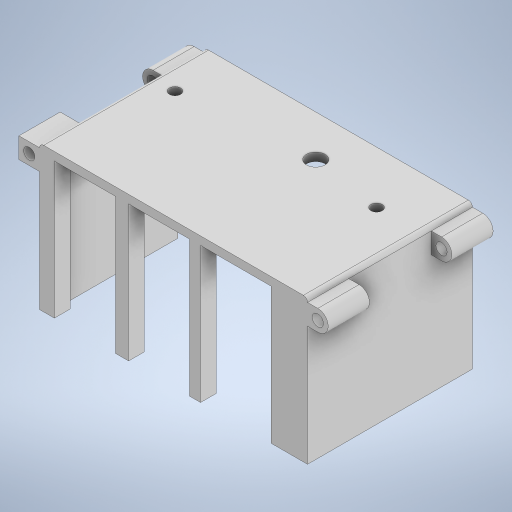
# Autodesk Inventor part: TOTAL
Saved by Autodesk Inventor 2023.1 (Build 271208000, 208)
## iProperties
Created: 2023-01-22
Part Number: TOTAL
Material: Generic
Document SubType Name: Modeling
Designer: liaar
Density: 1 g/cm^3
Appearance: Default
Author: liaar
Autodesk Inventor part; units mm, degrees
sketch "Sketch1" plane through (0, 0, 0) normal (0, 1, 0) x (-1, 0, 0)
  line L0 (0, 0) -> (-65, 0)
  line L1 (-65, 0) -> (-65, -121.25)
  line L2 (-65, -121.25) -> (0, -121.25)
  line L3 (0, -121.25) -> (0, 0)
  dimension "d0" = 121.25
  dimension "d1" = 65
  constraints: 8 end point, 2 parallel, 1 horizontal, 1 perpendicular
  measures "d0" distance of L0.end L1.end
  measures "d1" distance of L1.end L2.end
extrude "Extrusion1" add sketch "Sketch1" against normal blind 35
sketch "Sketch2" plane through (0, 0, 0) normal (0, 1, 0) x (1, 0, 0)
  line L0 (0, 0) -> (65, 0) projected
  line L1 (0, 121.25) -> (0, 0) projected
  circle A0 centre (54.45, 27.3) radius 1.35
  line L2 (65, 0) -> (65, 121.25) projected
  circle A1 centre (5.55, 27.3) radius 1.35
  circle A2 centre (5.55, 85.3) radius 1.5
  circle A3 centre (54.45, 85.3) radius 1.5
  line L3 (65, 121.25) -> (0, 121.25) projected
  dimension "d13" = 2.7
  dimension "d14" = 10.55
  dimension "d15" = 27.3
  dimension "d16" = 2.7
  dimension "d17" = 48.9
  dimension "d18" = 3
  dimension "d19" = 3
  dimension "d20" = 35.95
  constraints: 4 centre point, 2 horizontal alignment, 2 vertical alignment
  measures "d13" diameter of A0
  measures "d14" distance from line of L2 A0.centre
  measures "d15" distance from line of L0 A0.centre
  measures "d16" diameter of A1
  measures "d17" distance of A0.centre A1.centre
  measures "d18" diameter of A2
  measures "d19" diameter of A3
  measures "d20" distance from line of L3 A2.centre
extrude "Extrusion2" cut sketch "Sketch2" against normal through all contours A0 | A1 | A2 | A3
sketch "Sketch3" plane through (0, -35, 0) normal (0, -1, 0) x (1, 0, 0)
  line L0 (3.6, 0) -> (3.6, -3.8)
  line L1 (3.6, -3.8) -> (1.8, -3.8)
  line L2 (1.8, -3.8) -> (1.8, -23.85)
  line L3 (1.8, -30.25) -> (1.8, -82.3)
  line L4 (56.2, -112.3) -> (63.2, -112.3)
  line L5 (63.2, -112.3) -> (63.2, -55.25)
  line L6 (65, -121.25) -> (65, 0) projected
  line L7 (63.2, -23.85) -> (63.2, -3.8)
  line L8 (63.2, -3.8) -> (56.2, -3.8)
  line L9 (56.2, -3.8) -> (56.2, 0)
  line L10 (65, 0) -> (0, 0) projected
  line L11 (56.2, 0) -> (65, 0)
  line L12 (65, 0) -> (65, -121.25)
  line L13 (65, -121.25) -> (0, -121.25) projected
  line L14 (65, -121.25) -> (0, -121.25)
  line L15 (0, -121.25) -> (0, 0) projected
  line L16 (0, -121.25) -> (0, 0)
  line L17 (0, 0) -> (3.6, 0)
  line L18 (8.55, -119.45) -> (56.45, -119.45)
  line L19 (3.6, 0) -> (56.2, 0)
  line L20 (8.55, -119.45) -> (1.8, -119.45)
  line L21 (1.8, -119.45) -> (1.8, -82.3)
  line L22 (1.8, -30.25) -> (1.8, -23.85)
  line L23 (63.2, -23.85) -> (63.2, -55.25)
  line L24 (63.2, -112.3) -> (63.2, -119.45)
  line L25 (63.2, -119.45) -> (56.45, -119.45)
  line L26 (56.25, -23.85) -> (56.45, -23.85)
  line L27 (56.2, -23.85) -> (63.2, -23.85)
  line L28 (63.2, -55.25) -> (56.2, -55.25)
  line L29 (56.45, -30.25) -> (56.25, -30.25)
  dimension "d35" = 3.8
  dimension "d36" = 3.6
  dimension "d37" = 1.8
  dimension "d44" = 1.8
  dimension "d46" = 8.95
  dimension "d47" = 1.8
  dimension "d48" = 57.05
  dimension "d50" = 20.05
  dimension "d51" = 3.8
  dimension "d52" = 8.8
  constraints: 52 end point, 9 perpendicular, 8 point on line, 5 collinear, 2 parallel, 2 vertical, 1 coincident, 1 horizontal
  measures "d35" distance of L0.start L0.end
  measures "d36" distance between parallel lines of L15 L0
  measures "d37" distance between parallel lines of L15 L2
  measures "d44" distance between parallel lines of L14 L18
  measures "d46" distance between parallel lines of L13 L4
  measures "d47" distance between parallel lines of L6 L5
  measures "d48" distance of L4.end L5.end
  measures "d50" distance of L7.start L7.end
  measures "d51" distance of L8.end L9.end
  measures "d52" distance of L6.end L9.end
extrude "Extrusion3" cut sketch "Sketch3" against normal blind 33 contours L10 L9 L8 L7 L23 L5 L24 L25 L18 L20 L21 L3 L22 L2 L1 L0
sketch "Sketch4" plane through (0, -2, 0) normal (0, -1, 0) x (1, 0, 0)
  line L0 (0, 0) -> (65, 0) projected
  line L1 (18.4, 0) -> (21.6, 0)
  line L2 (21.6, 0) -> (21.6, -3.8)
  line L3 (21.6, -3.8) -> (18.4, -3.8)
  line L4 (18.4, -3.8) -> (18.4, 0)
  line L5 (39.05, 0) -> (36.4, 0)
  line L6 (36.4, 0) -> (36.4, -3.8)
  line L7 (36.4, -3.8) -> (39.05, -3.8)
  line L8 (39.05, -3.8) -> (39.05, 0)
  line L9 (3.6, -3.8) -> (3.6, 0) projected
  dimension "d55" = 14.8
  dimension "d56" = 3.2
  dimension "d57" = 2.65
  dimension "d58" = 14.8
  constraints: 16 end point, 4 parallel, 3 point on line, 2 horizontal, 2 perpendicular, 1 horizontal alignment
  measures "d55" distance between parallel lines of L4 L9
  measures "d56" distance between parallel lines of L2 L4
  measures "d57" distance between parallel lines of L8 L6
  measures "d58" distance between parallel lines of L6 L2
extrude "Extrusion4" add sketch "Sketch4" along normal up to surface (33 mm away)
ref_plane "Work Plane1" through (20, -2, -3.8) normal (-1, 0, 0) x (0, 0, 1)
ref_plane "Work Plane2" through (37.725, -2, 0) normal (1, 0, 0) x (0, 0, -1)
sketch "Sketch18" plane through (0, 0, -121.25) normal (-1, 0, 0) x (0, 0, 1)
  line L0 (0, -35) -> (121.25, -35) projected
  line L1 (38.95, -35) -> (48.2, -35)
  line L2 (48.2, -35) -> (48.2, -30.35)
  line L3 (48.2, -30.35) -> (38.95, -30.35)
  line L4 (38.95, -30.35) -> (38.95, -35)
  line L5 (54.35, -35) -> (62.15, -35)
  line L6 (62.15, -35) -> (62.15, -30.35)
  line L7 (62.15, -30.35) -> (54.35, -30.35)
  line L8 (54.35, -30.35) -> (54.35, -35)
  line L9 (67.85, -35) -> (75.65, -35)
  line L10 (75.65, -35) -> (75.65, -30.35)
  line L11 (75.65, -30.35) -> (67.85, -30.35)
  line L12 (67.85, -30.35) -> (67.85, -35)
  line L13 (83.005, -35) -> (89.505, -35)
  line L14 (89.505, -35) -> (89.505, -29)
  line L15 (89.505, -29) -> (83.005, -29)
  line L16 (83.005, -29) -> (83.005, -35)
  arc A0 (89.505, -29) -> (83.005, -29) centre (86.255, -29) ccw
  line L17 (0, 0) -> (0, -35) projected
  point P0 (121.25, 0)
  point P1 (54.35, -32.675)
  point P2 (48.2, -32.675)
  point P3 (75.65, -32.675)
  point P4 (43.575, -35)
  point P5 (62.15, -35)
  dimension "d148" = 38.95
  dimension "d149" = 9.25
  dimension "d150" = 6.15
  dimension "d151" = 5.7
  dimension "d152" = 7.8
  dimension "d153" = 7.8
  dimension "d154" = 7.355
  dimension "d155" = 6.5
  dimension "d156" = 6
  dimension "d157" = 4.65
  constraints: 32 end point, 8 parallel, 6 point on line, 4 horizontal, 4 midpoint, 4 perpendicular, 2 point on circle, 2 tangent, 1 centre point
  measures "d148" distance between parallel lines of L17 L4
  measures "d149" distance between parallel lines of L2 L4
  measures "d150" distance of point (54.35, -32.675) point (48.2, -32.675)
  measures "d151" distance between parallel lines of L12 L6
  measures "d152" distance of L6.end L7.end
  measures "d153" distance of L10.end L11.end
  measures "d154" distance from line of L16 point (75.65, -32.675)
  measures "d155" distance of L13.start L13.end
  measures "d156" distance between parallel lines of L13 L15
  measures "d157" distance from line of point (43.575, -35) L3
extrude "Extrusion17" cut sketch "Sketch18" against normal up to surface (1.8 mm away)
ref_plane "Work Plane6" through (0, 0, -41.15) normal (0, 0, 1) x (1, 0, 0)
sketch "Sketch22" plane through (65, 0, -121.25) normal (0, 0, -1) x (-1, 0, 0)
  line L0 (1.8, -1.8) -> (63.2, -1.8)
  line L1 (63.2, -1.8) -> (63.2, -25)
  line L2 (63.2, -25) -> (1.8, -25)
  line L3 (1.8, -25) -> (1.8, -1.8)
  line L4 (0, 0) -> (0, -35) projected
  line L5 (65, 0) -> (65, -35) projected
  line L6 (0, 0) -> (65, 0) projected
  line L7 (65, -35) -> (0, -35) projected
  dimension "d172" = 1.8
  dimension "d173" = 1.8
  dimension "d174" = 1.8
  dimension "d175" = 10
  constraints: 8 end point, 2 parallel, 1 horizontal, 1 perpendicular
  measures "d172" distance between parallel lines of L4 L3
  measures "d173" distance between parallel lines of L5 L1
  measures "d174" distance between parallel lines of L6 L0
  measures "d175" distance between parallel lines of L7 L2
extrude "Extrusion21" cut sketch "Sketch22" against normal blind 7.5 contours L0 L1 L2 L3
sketch "Sketch23" plane through (1.8, -35, -3.8) normal (1, 0, 0) x (0, 0, -1)
  line L0 (36.2, 12) -> (55.05, 12)
  line L1 (55.05, 12) -> (55.05, 10)
  line L2 (55.05, 10) -> (36.2, 10)
  line L3 (36.2, 10) -> (36.2, 12)
  line L4 (-3.8, 35) -> (-3.8, 0) projected
  line L5 (-3.8, 0) -> (27.945, 0) projected
  line L6 (37.35, 42) -> (37.35, -7) projected
  point P0 (-3.8, 30)
  dimension "d178" = 2
  dimension "d180" = 40
  dimension "d181" = 10
  dimension "d184" = 18.85
  constraints: 8 end point, 2 parallel, 1 horizontal, 1 perpendicular
  measures "d178" distance between parallel lines of L0 L2
  measures "d180" distance between parallel lines of L4 L3
  measures "d181" distance between parallel lines of L2 L5
  measures "d184" distance of L1.end L2.end
extrude "Extrusion22" add sketch "Sketch23" along normal blind 7.5
fillet "Fillet2" radius 1 5 edges at (0, 0, -60.625) (32.5, 0, -121.25) (0, -17.5, -121.25) (65, -17.5, -121.25) (65, 0, -60.625)
fillet "Fillet3" radius 1 1 edges at (32.5, -25, -119.45)
sketch "Sketch26" plane through (0, 0, 0) normal (0, 1, 0) x (1, 0, 0)
  line L0 (37, 140.8638) -> (37, -4.3426) construction
  line L1 (0, 120.25) -> (0, 0) projected
  circle A0 centre (37, 30) radius 2.25
  circle A1 centre (37, 43) radius 2.25
  circle A2 centre (37, 56) radius 2.25
  circle A3 centre (37, 69) radius 2.25
  circle A4 centre (37, 82) radius 2.25
  line L2 (1, 0) -> (64, 0) projected
  point P0 (0, 33.65)
  point P1 (0, 7.5)
  dimension "d192" = 37
  dimension "d194" = 4.5
  dimension "d195" = 13
  dimension "d196" = 13
  dimension "d197" = 13
  dimension "d198" = 13
  dimension "d201" = 30
  constraints: 5 centre point, 5 point on line, 4 equal radius, 2 end point, 1 vertical
  measures "d192" distance between parallel lines of L1 L0
  measures "d194" diameter of A0
  measures "d195" distance of A0.centre A1.centre
  measures "d196" distance of A2.centre A1.centre
  measures "d197" distance of A3.centre A2.centre
  measures "d198" distance of A4.centre A3.centre
  measures "d201" distance from line of L2 A0.centre
extrude "Extrusion23" cut sketch "Sketch26" against normal up to surface (2 mm away)
ref_plane "Work Plane8" through (56.2, -35, -40) normal (0, 0, 1) x (1, 0, 0)
sketch "Sketch27" plane through (56.2, -35, -40) normal (0, 0, 1) x (1, 0, 0)
  line L0 (-71.0264, 49.2506) -> (25.2733, 49.2506)
  line L1 (25.2733, 49.2506) -> (25.2733, -11.0626)
  line L2 (25.2733, -11.0626) -> (-71.0264, -11.0626)
  line L3 (-71.0264, -11.0626) -> (-71.0264, 49.2506)
  point P0 (-56.2, 35)
  constraints: 8 end point, 2 parallel, 1 horizontal, 1 perpendicular
extrude "Extrusion24" cut sketch "Sketch27" against normal up to surface (81.25 mm away)
sketch "Sketch28" plane through (56.2, -35, 0) normal (0, 0, 1) x (1, 0, 0)
  line L0 (8.8, 34) -> (8.8, 0) projected
  line L1 (8.8, 34) -> (13.8, 34)
  line L2 (13.8, 34) -> (13.8, 29)
  line L3 (13.8, 29) -> (8.8, 29)
  line L4 (8.8, 29) -> (8.8, 34)
  line L5 (-56.2, 34) -> (-56.2, 0) projected
  line L6 (-56.2, 34) -> (-61.2, 34)
  line L7 (-61.2, 34) -> (-61.2, 29)
  line L8 (-61.2, 29) -> (-56.2, 29)
  line L9 (-56.2, 29) -> (-56.2, 34)
  circle A0 centre (-58.7, 31.5) radius 1.35
  circle A1 centre (11.3, 31.5) radius 1.35
  point P0 (-56.2, 35)
  dimension "d205" = 5
  dimension "d206" = 5
  dimension "d207" = 2.7
  dimension "d208" = 2.7
  dimension "d209" = 2.5
  dimension "d210" = 2.5
  dimension "d211" = 2.5
  dimension "d212" = 2.5
  constraints: 16 end point, 4 parallel, 4 perpendicular, 2 centre point, 2 horizontal
  measures "d205" distance of L0.start L1.end
  measures "d206" distance of L5.start L6.end
  measures "d207" diameter of A0
  measures "d208" diameter of A1
  measures "d209" distance from line of L1 A1.centre
  measures "d210" distance from line of L2 A1.centre
  measures "d211" distance from line of L8 A0.centre
  measures "d212" distance from line of L7 A0.centre
extrude "Extrusion25" add sketch "Sketch28" against normal blind 10
sketch "Sketch29" plane through (56.2, -35, -40) normal (0, 0, -1) x (-1, 0, 0)
  line L0 (56.2, 29) -> (56.2, 34) projected
  line L1 (61.2, 29) -> (56.2, 29) projected
  line L2 (56.2, 34) -> (61.2, 34)
  line L3 (61.2, 34) -> (61.2, 29)
  line L4 (61.2, 29) -> (56.2, 29)
  line L5 (56.2, 29) -> (56.2, 34)
  circle A0 centre (58.7, 31.5) radius 1.35 projected
  circle A1 centre (58.7, 31.5) radius 1.35
  line L6 (-13.8, 29) -> (-13.8, 34) projected
  line L7 (-8.8, 34) -> (-13.8, 34)
  line L8 (-13.8, 34) -> (-13.8, 29)
  line L9 (-13.8, 29) -> (-8.8, 29)
  line L10 (-8.8, 29) -> (-8.8, 34)
  circle A2 centre (-11.3, 31.5) radius 1.35 projected
  circle A3 centre (-11.3, 31.5) radius 1.35
  point P0 (56.2, 35)
  constraints: 16 end point, 4 parallel, 2 centre point, 2 coincident, 2 horizontal, 2 perpendicular
extrude "Extrusion26" add sketch "Sketch29" against normal blind 10
full round fillet "Full Round Fillet5" first side at (-1.6667, -1, -33.3333) centre faces at (-5, -4.3333, -36.6667) second side at (-1.6667, -6, -36.6667)
full round fillet "Full Round Fillet6" first side at (68.3333, -1, -3.3333) centre faces at (70, -4.3333, -3.3333) second side at (66.6667, -6, -3.3333)
full round fillet "Full Round Fillet7" first side at (66.6667, -1, -36.6667) centre faces at (70, -2.6667, -36.6667) second side at (68.3333, -6, -36.6667)
body "Solid1"
